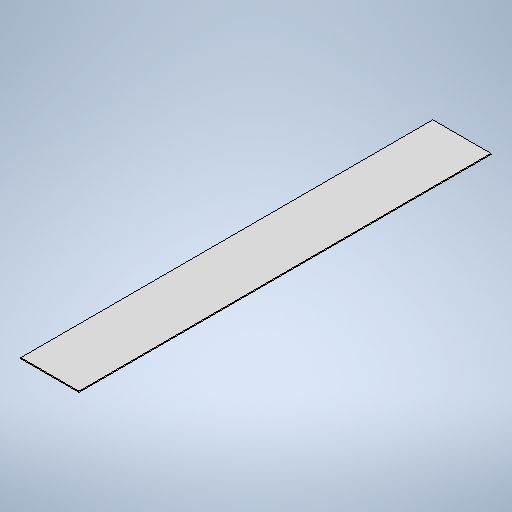
# Autodesk Inventor part: MNT-CDF-603 CAP
Saved by Autodesk Inventor 2025 (Build 290162010, 162A)
## iProperties
Created: 2025-01-16
Part Number: MNT-CDF-603 CAP
Material: Stainless Steel
Document SubType Name: Sheet Metal
Designer: pokla
Density: 8 g/cm^3
Sheet Metal Rule: AISI304 2mm Die16
Appearance: Default
Author: pokla
Autodesk Inventor part; units mm, degrees
ref_plane "YZ Plane" through (0, 0, 0) normal (1, 0, 0) x (0, 1, 0)
ref_plane "XZ Plane" through (0, 0, 0) normal (0, 1, 0) x (-1, 0, 0)
ref_plane "XY Plane" through (0, 0, 0) normal (0, 0, 1) x (1, 0, 0)
sketch "Sketch1" plane through (0, 0, 0) normal (0, 0, 1) x (1, 0, 0)
  line L0 (-60, 425.027) -> (60, 425.027)
  line L1 (60, 425.027) -> (60, -425.027)
  line L2 (60, -425.027) -> (-60, -425.027)
  line L3 (-60, -425.027) -> (-60, 425.027)
  line L4 (-60, 425.027) -> (60, -425.027) construction
  point P0 (0, 0)
  point P1 (0, 0)
  dimension "d0" = 120
  dimension "d1" = 850.054
  measures "d0" distance of L0.start L0.end
  measures "d1" distance of L2.end L0.start
extrude "Plate1" add sketch "Sketch1" along normal blind 2
sketch "Sketch2" plane through (60, -425.027, 0) normal (1, 0, 0) x (0, 0, -1)
  line L0 (0, 0) -> (0, 850.054) projected
  line L1 (0, 850.054) -> (-2, 849.5553)
  line L2 (-2, 850.054) -> (-2, 0) projected
  line L3 (0, 850.054) -> (-2, 850.054) projected
  point P0 (0, 425.027)
  dimension "d4" = 14
  constraints: 2 end point, 1 point on line
  measures "d4" angle of L3 L1
extrude "Extrusion1" cut sketch "Sketch2" against normal through all
equation "\"d2\" = Thickness"
equation "\"BendReliefWidth\" = Thickness"
equation "\"BendReliefDepth\" = 0.5 * Thickness"
equation "\"CornerReliefSize\" = 4 * Thickness"
equation "\"MinimumRemnant\" = 2 * Thickness"
equation "\"TransitionRadius\" = BendRadius"
equation "\"JacobiRadiusSize\" = BendRadius"
equation "\"GapSize\" = Thickness"
equation "\"Thickness\" = 2"
equation "\"BendRadius\" = 2.75"
body "Solid1"
